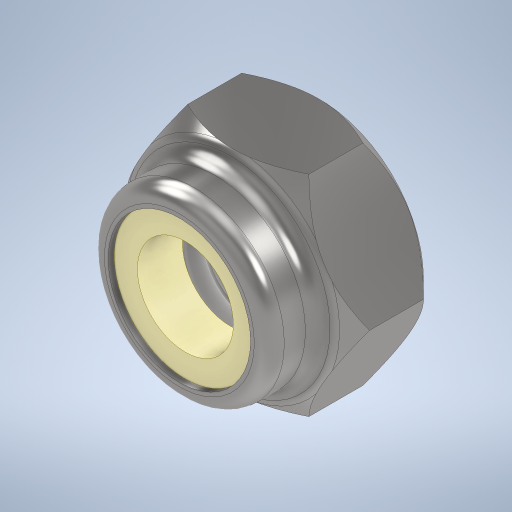
# Autodesk Inventor part: M4 LOCKNUT
Saved by Autodesk Inventor 2024 (Build 280153000, 153)
## iProperties
Created: 2024-09-05
Part Number: M4 LOCKNUT
Material: Stainless Steel
Document SubType Name: Modeling
Designer: Ishaan
Density: 8 g/cm^3
Appearance: Semi-Polished
Author: Ishaan
Autodesk Inventor part; units mm, degrees
ref_plane "YZ Plane" through (0, 0, 0) normal (1, 0, 0) x (0, 1, 0)
ref_plane "XZ Plane" through (0, 0, 0) normal (0, 1, 0) x (-1, 0, 0)
ref_plane "XY Plane" through (0, 0, 0) normal (0, 0, 1) x (1, 0, 0)
sketch "Sketch1" plane through (0, 0, 0) normal (0, 0, 1) x (1, 0, 0)
  circle A0 centre (0, 0) radius 4.041452
  line L0 (-2.020726, 3.5) -> (2.020726, 3.5)
  line L1 (2.020726, 3.5) -> (4.041452, 0)
  line L2 (4.041452, 0) -> (2.020726, -3.5)
  line L3 (2.020726, -3.5) -> (-2.020726, -3.5)
  line L4 (-2.020726, -3.5) -> (-4.041452, 0)
  line L5 (-4.041452, 0) -> (-2.020726, 3.5)
  point P0 (-4.041452, 0)
  point P1 (-4.041452, 0)
  point P2 (4.041452, 0)
  point P3 (4.041452, 0)
  dimension "d0" = 7
  constraints: 12 end point, 2 coincident, 1 horizontal, 16 other
  measures "d0" distance between parallel lines of L3 L0
extrude "Extrusion1" add sketch "Sketch1" along normal blind 3
chamfer "Chamfer1" distance 0.6 angle 45 2 edges at (-4.0415, 0, 0) (-4.0415, 0, 3)
extrude "Extrusion2" cut sketch "Sketch1" along normal through all contours L1 A0 | A0 L2 | L0 A0 | A0 L3 | L5 A0 | A0 L4
sketch "Sketch2" plane through (0, 0, 3) normal (0, 0, 1) x (1, 0, 0)
  circle A0 centre (0, 0) radius 3.441452
  circle A1 centre (0, 0) radius 3
  dimension "d9" = 6
  constraints: 1 centre point, 1 coincident
  measures "d9" diameter of A1
extrude "Extrusion3" add sketch "Sketch2" along normal blind 1.7 contours A1
fillet "Fillet1" radius 0.5 3 edges at (-3, 0, 3) (-3.4415, 0, 3) (-3, 0, 4.7)
sketch "Sketch3" plane through (0, 0, 4.7) normal (0, 0, 1) x (1, 0, 0)
  circle A0 centre (0, 0) radius 2.375
  dimension "d13" = 4.75
  constraints: 1 centre point, 1 coincident
  measures "d13" diameter of A0
extrude "Extrusion4" cut sketch "Sketch3" against normal blind 1.7
sketch "Sketch4" plane through (0, 0, 3) normal (0, 0, 1) x (1, 0, 0)
  circle A0 centre (0, 0) radius 2.375 projected
extrude "Extrusion5" add sketch "Sketch4" along normal blind 1.5 separate body
sketch "Sketch5" plane through (0, 0, 4.5) normal (0, 0, 1) x (1, 0, 0)
  circle A0 centre (0, 0) radius 2.375 projected
  constraints: 1 coincident
hole "Hole1" at (0, 0, 4.5) direction (0, 0, -1) diameter 3.242 end through all bodies 1 thread size "M4x0.7" class "6H" standard "ANSI Metric M Profile"
sketch "Sketch6" plane through (0, 0, 3) normal (0, 0, -1) x (-1, 0, 0)
  circle A0 centre (0, 0) radius 1.621 projected
  constraints: 1 coincident
hole "Hole2" at (0, 0, 3) direction (0, 0, 1) diameter 3.2 end through all bodies 2
chamfer "Chamfer2" distance 0.25 angle 45 1 edges at (0, 1.621, 0)
body "Solid1"
